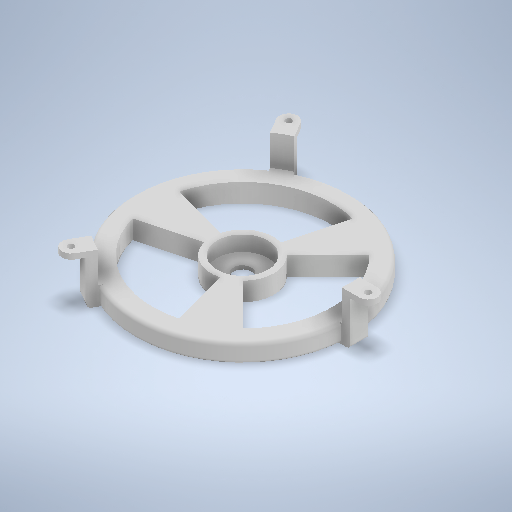
# Autodesk Inventor part: MechSwitch_DielecTopV3
Saved by Autodesk Inventor 2025.1 (Build 291241000, 241)
## iProperties
Created: 2026-04-20
Part Number: MechSwitch_DielecTopV3
Material: Generic
Document SubType Name: Modeling
Designer: ryand
Density: 1 g/cm^3
Appearance: Default
Author: ryand
Autodesk Inventor part; units mm, degrees
ref_plane "YZ Plane" through (0, 0, 0) normal (1, 0, 0) x (0, 1, 0)
ref_plane "XZ Plane" through (0, 0, 0) normal (0, 1, 0) x (-1, 0, 0)
ref_plane "XY Plane" through (0, 0, 0) normal (0, 0, 1) x (1, 0, 0)
sketch "Sketch1" plane through (0, 0, 0) normal (0, 1, 0) x (-1, 0, 0)
  arc A0 (48.2963, 12.941) -> (48.2963, -12.941) centre (0, 0) ccw
  line L0 (16.9037, -4.5293) -> (48.2963, -12.941)
  line L1 (0, 0) -> (50, 0) construction
  line L2 (16.9037, 4.5293) -> (48.2963, 12.941)
  line L3 (0, 0) -> (50, 0) construction
  line L4 (-12.3744, 12.3744) -> (-35.3553, 35.3553)
  line L5 (-4.5293, 16.9037) -> (-12.941, 48.2963)
  line L6 (-4.5293, -16.9037) -> (-12.941, -48.2963)
  line L7 (-12.3744, -12.3744) -> (-35.3553, -35.3553)
  arc A1 (16.9037, 4.5293) -> (-4.5293, 16.9037) centre (0, 0) ccw
  arc A2 (-12.3744, 12.3744) -> (-12.3744, -12.3744) centre (0, 0) ccw
  arc A3 (-4.5293, -16.9037) -> (16.9037, -4.5293) centre (0, 0) ccw
  line L8 (-65, 5) -> (-65, -5)
  line L9 (-65, 5) -> (-59.7913, 5)
  line L10 (-65, -5) -> (-59.7913, -5)
  line L11 (28.1699, -58.7917) -> (25.5655, -54.2808)
  line L12 (28.1699, -58.7917) -> (36.8301, -53.7917)
  line L13 (36.8301, -53.7917) -> (34.2258, -49.2808)
  line L14 (36.8301, 53.7917) -> (34.2258, 49.2808)
  line L15 (36.8301, 53.7917) -> (28.1699, 58.7917)
  line L16 (28.1699, 58.7917) -> (25.5655, 54.2808)
  arc A4 (34.2258, -49.2808) -> (34.2258, 49.2808) centre (0, 0) ccw
  arc A5 (25.5655, 54.2808) -> (-59.7913, 5) centre (0, 0) ccw
  arc A6 (-59.7913, -5) -> (25.5655, -54.2808) centre (0, 0) ccw
  dimension "d1" = 100
  dimension "d3" = 15
  dimension "d5" = 15
  dimension "d14" = 360
  dimension "d16" = 17.5
  dimension "d17" = 24.7487
  dimension "d19" = 10
  dimension "d21" = 65
  dimension "d24" = 360
  constraints: 34 end point, 14 point on circle, 7 centre point, 3 horizontal, 2 coincident, 1 parallel, 41 other
  measures "d1" diameter of A0
  measures "d3" angle of L0 L1
  measures "d5" angle of L3 L2
  measures "d16" radius of A1
  measures "d17" distance of L2.start L5.start
  measures "d19" distance of L8.end L8.start
  measures "d21" distance from line of point (0, 0) L8
extrude "Extrusion1" add sketch "Sketch1" along normal blind 10.4
sketch "Sketch2" plane through (0, 10.4, 0) normal (0, 1, 0) x (1, 0, 0)
  arc A0 (60.293, -5) -> (60.293, 5) centre (0, 0) ccw
  line L0 (65, -5) -> (65, 5) projected
  line L1 (65, -5) -> (60.293, -5)
  line L2 (60.293, 5) -> (65, 5)
  line L3 (65, 5) -> (65, -5)
  arc A1 (-25.8164, 54.7153) -> (-34.4766, 49.7153) centre (0, 0) ccw
  line L4 (-28.1699, 58.7917) -> (-25.8164, 54.7153)
  line L5 (-34.4766, 49.7153) -> (-36.8301, 53.7917)
  line L6 (-36.8301, 53.7917) -> (-28.1699, 58.7917)
  arc A2 (-34.4766, -49.7153) -> (-25.8164, -54.7153) centre (0, 0) ccw
  line L7 (-36.8301, -53.7917) -> (-34.4766, -49.7153)
  line L8 (-25.8164, -54.7153) -> (-28.1699, -58.7917)
  line L9 (-28.1699, -58.7917) -> (-36.8301, -53.7917)
  dimension "d28" = 121
  dimension "d29" = 10
  dimension "d33" = 360
  constraints: 18 end point, 6 point on circle, 3 centre point, 1 coincident, 1 horizontal, 1 parallel, 28 other
  measures "d28" diameter of A0
  measures "d29" distance between parallel lines of L1 L2
extrude "Extrusion2" add sketch "Sketch2" along normal blind 17.1
sketch "Sketch3" plane through (0, 10.4, 0) normal (0, 1, 0) x (1, 0, 0)
  circle A0 centre (0, 0) radius 14.15
  dimension "d37" = 28.3
  constraints: 1 centre point, 1 coincident
  measures "d37" diameter of A0
extrude "Extrusion3" cut sketch "Sketch3" against normal blind 8.4
sketch "Sketch4" plane through (0, 2, 0) normal (0, 1, 0) x (1, 0, 0)
  circle A0 centre (0, 0) radius 5
  dimension "d40" = 10
  constraints: 1 centre point, 1 coincident
  measures "d40" diameter of A0
extrude "Extrusion4" cut sketch "Sketch4" against normal blind 2
sketch "Sketch5" plane through (0, 27.5, 0) normal (0, 1, 0) x (1, 0, 0)
  circle A0 centre (70, 0) radius 1.75
  line L0 (65, -5) -> (65, 5) projected
  line L1 (65, 5) -> (70, 5)
  line L2 (65, -5) -> (70, -5)
  line L3 (65, 5) -> (65, -5)
  arc A1 (70, -5) -> (70, 5) centre (70, 0) ccw
  line L4 (70, -5) -> (65, -5)
  circle A2 centre (-35, 60.6218) radius 1.75
  line L5 (-36.8301, 53.7917) -> (-39.3301, 58.1218)
  line L6 (-28.1699, 58.7917) -> (-30.6699, 63.1218)
  line L7 (-36.8301, 53.7917) -> (-28.1699, 58.7917)
  arc A3 (-30.6699, 63.1218) -> (-39.3301, 58.1218) centre (-35, 60.6218) ccw
  line L8 (-30.6699, 63.1218) -> (-28.1699, 58.7917)
  circle A4 centre (-35, -60.6218) radius 1.75
  line L9 (-28.1699, -58.7917) -> (-30.6699, -63.1218)
  line L10 (-36.8301, -53.7917) -> (-39.3301, -58.1218)
  line L11 (-28.1699, -58.7917) -> (-36.8301, -53.7917)
  arc A5 (-39.3301, -58.1218) -> (-30.6699, -63.1218) centre (-35, -60.6218) ccw
  line L12 (-39.3301, -58.1218) -> (-36.8301, -53.7917)
  point P0 (0, 0)
  point P1 (62.6465, -5)
  dimension "d43" = 3.5
  dimension "d44" = 70
  dimension "d45" = 5
  dimension "d48" = 360
  constraints: 24 end point, 6 centre point, 6 point on circle, 3 coincident, 3 equal length, 2 horizontal, 1 tangent, 37 other
  measures "d43" diameter of A0
  measures "d44" distance of point (0, 0) A0.centre
  measures "d45" vertical distance of point (62.647, -5) A0.centre
extrude "Extrusion5" add sketch "Sketch5" against normal blind 3
fillet "Fillet1" radius 2 3 edges at (-32.5, 0, -56.2917) (-32.5, 0, 56.2917) (65, 0, 0)
fillet "Fillet2" radius 2 6 edges at (-60, 0, 0) (30, 0, -51.9615) (30, 0, 51.9615) (30, 10.4, 51.9615) (30, 10.4, -51.9615) (-60, 10.4, 0)
body "Solid1"
